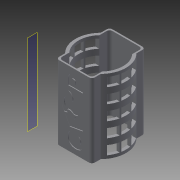
# Autodesk Inventor part: Lattice
Saved by Autodesk Inventor 2013 (Build 170138000, 138)
## iProperties
Created: 2014-07-03
Part Number: Lattice
Material: Genérico
Document SubType Name: Chapa
Designer: Administrador
Density: 1 g/cm^3
Sheet Metal Rule: Por defecto_mm
Author: Administrador
Autodesk Inventor part; units mm, degrees
ref_plane "YZ Plane" through (0, 0, 0) normal (1, 0, 0) x (0, 1, 0)
ref_plane "XZ Plane" through (0, 0, 0) normal (0, 1, 0) x (-1, 0, 0)
ref_plane "XY Plane" through (0, 0, 0) normal (0, 0, 1) x (1, 0, 0)
sketch "Boceto2" plane through (0, 0, 0) normal (0, 0, 1) x (1, 0, 0)
  line L0 (-11.1, -17.1) -> (11.1, -17.1)
  line L1 (11.1, 17.1) -> (-11.1, 17.1)
  line L2 (-11.1, -17.1) -> (11.1, 17.1) construction
  line L3 (11.1, -17.1) -> (-11.1, 17.1) construction
  arc A0 (-12.1, 12.083) -> (-12.1, -12.083) centre (0, 0) ccw
  arc A1 (12.1, -12.083) -> (12.1, 12.083) centre (0, 0) ccw
  line L4 (11.1, -17.1) -> (11.1, -13.0077)
  line L5 (11.1, 13.0077) -> (11.1, 17.1)
  line L6 (-11.1, 17.1) -> (-11.1, 13.0077)
  line L7 (-11.1, -13.0077) -> (-11.1, -17.1)
  line L8 (-44.1235, -12.996) -> (-27.2515, -12.996)
  line L9 (-27.2515, 12.996) -> (-44.1235, 12.996)
  line L10 (-44.1235, -12.996) -> (-27.2515, 12.996) construction
  line L11 (-27.2515, -12.996) -> (-44.1235, 12.996) construction
  arc A2 (-44.1235, 9.8858) -> (-44.1235, -9.8858) centre (-35.6875, 0) ccw
  arc A3 (-27.2515, -9.8858) -> (-27.2515, 9.8858) centre (-35.6875, 0) ccw
  line L12 (-27.2515, -12.996) -> (-27.2515, -9.8858)
  line L13 (-27.2515, 9.8858) -> (-27.2515, 12.996)
  line L14 (-44.1235, 12.996) -> (-44.1235, 9.8858)
  line L15 (-44.1235, -9.8858) -> (-44.1235, -12.996)
  line L16 (-12.1, -18.1) -> (12.1, -18.1)
  line L17 (12.1, 18.1) -> (-12.1, 18.1)
  line L18 (-12.1, -18.1) -> (12.1, 18.1) construction
  line L19 (12.1, -18.1) -> (-12.1, 18.1) construction
  line L20 (-12.1, 18.1) -> (-12.1, 12.083)
  line L21 (-12.1, -12.083) -> (-12.1, -18.1)
  line L22 (12.1, -18.1) -> (12.1, -12.083)
  line L23 (12.1, 12.083) -> (12.1, 18.1)
  arc A4 (-8.2215, 12.6656) -> (-8.392, 12.5533) centre (0, 0) ccw
  arc A5 (8.392, 12.5533) -> (8.2215, 12.6656) centre (0, 0) ccw
  arc A6 (-11.1, 10.2372) -> (-11.1, -10.2372) centre (0, 0) ccw
  arc A7 (-8.392, -12.5533) -> (-8.2215, -12.6656) centre (0, 0) ccw
  arc A8 (8.2215, -12.6656) -> (8.392, -12.5533) centre (0, 0) ccw
  arc A9 (11.1, -10.2372) -> (11.1, 10.2372) centre (0, 0) ccw
  line L24 (11.1, 12.996) -> (11.1, 10.2372)
  line L25 (11.1, -10.2372) -> (11.1, -12.996)
  line L26 (-11.1, 12.996) -> (-11.1, 10.2372)
  line L27 (-11.1, -10.2372) -> (-11.1, -12.996)
  dimension "d4" = 22.2
  dimension "d5" = 34.2
  dimension "d6" = 16.872
  dimension "d7" = 25.992
  dimension "d9" = 24.2
  dimension "d10" = 36.2
  constraints: 56 end point, 20 point on circle, 15 parallel, 10 centre point, 8 point on line, 6 midpoint, 6 perpendicular, 3 horizontal
  measures "d4" distance of L1.end L1.start
  measures "d5" distance of L1.start L0.end
  measures "d6" distance of L9.end L9.start
  measures "d7" distance of L9.start L8.end
  measures "d9" distance of L17.end L17.start
  measures "d10" distance of L17.start L16.end
extrude "Extrusión1" add sketch "Boceto2" along normal blind 50 contours L20 L17 L23 A1 L22 L16 L21 A0
sketch "Boceto3" plane through (0, 0, 0) normal (0, 0, -1) x (-1, 0, 0)
  line L0 (24.6329, -16.764) -> (46.8329, -16.764)
  line L1 (46.8329, 17.436) -> (24.6329, 17.436)
  line L2 (46.8329, -16.764) -> (46.8329, -12.6716)
  line L3 (46.8329, 13.3437) -> (46.8329, 17.436)
  line L4 (24.6329, 17.436) -> (24.6329, 13.3437)
  line L5 (24.6329, -12.6716) -> (24.6329, -16.764)
  arc A0 (24.6329, 10.5732) -> (24.6329, -9.9011) centre (35.7329, 0.336) ccw
  arc A1 (46.8329, -9.9011) -> (46.8329, 10.5732) centre (35.7329, 0.336) ccw
  line L6 (46.8329, 13.332) -> (46.8329, 10.5732)
  line L7 (46.8329, -9.9011) -> (46.8329, -12.66)
  line L8 (24.6329, 13.332) -> (24.6329, 10.5732)
  line L9 (24.6329, -9.9011) -> (24.6329, -12.66)
  line L10 (-11.1, 17.1) -> (11.1, 17.1)
  line L11 (11.1, -17.1) -> (-11.1, -17.1)
  line L12 (-11.1, 17.1) -> (11.1, -17.1) construction
  line L13 (11.1, 17.1) -> (-11.1, -17.1) construction
  line L14 (11.1, 17.1) -> (11.1, 10.2372)
  line L15 (11.1, -10.2372) -> (11.1, -17.1)
  arc A2 (-11.1, 10.2372) -> (-11.1, -10.2372) centre (0, 0) ccw
  arc A3 (11.1, -10.2372) -> (11.1, 10.2372) centre (0, 0) ccw
  line L16 (-11.1, -17.1) -> (-11.1, -10.2372)
  line L17 (-11.1, 10.2372) -> (-11.1, 17.1)
  dimension "d13" = 22.2
  dimension "d14" = 34.2
  dimension "d15" = 22.2
  dimension "d16" = 34.2
  constraints: 36 end point, 10 parallel, 8 point on circle, 4 centre point, 4 perpendicular, 2 horizontal, 2 midpoint
  measures "d13" distance of L1.end L1.start
  measures "d14" distance of L1.start L0.end
  measures "d15" distance of L11.start L11.end
  measures "d16" distance of L10.end L11.start
extrude "Extrusión2" cut sketch "Boceto3" against normal through all
ref_plane "Plano de trabajo1" through (-31.35, -18.1, 0) normal (-1, 0, 0) x (0, 0, 1)
sketch "Boceto4" plane through (-31.35, -18.1, 0) normal (-1, 0, 0) x (0, 0, 1)
  line L0 (0, 6.017) -> (0, 30.183) projected
  line L1 (0, 36.2) -> (0, 30.183) projected
  line L2 (0, 30.183) -> (50, 30.183) projected
  line L3 (0, 6.017) -> (50, 6.017) projected
  line L4 (50, 6.017) -> (50, 30.183) projected
  line L5 (2.0442, 28.2647) -> (8.0442, 28.2647)
  line L6 (8.0442, 28.2647) -> (8.0442, 22.2647)
  line L7 (8.0442, 22.2647) -> (2.0442, 22.2647)
  line L8 (2.0442, 22.2647) -> (2.0442, 28.2647)
  line L9 (12.0442, 28.2647) -> (18.0442, 28.2647)
  line L10 (18.0442, 28.2647) -> (18.0442, 22.2647)
  line L11 (18.0442, 22.2647) -> (12.0442, 22.2647)
  line L12 (12.0442, 22.2647) -> (12.0442, 28.2647)
  line L13 (22.0442, 28.2647) -> (28.0442, 28.2647)
  line L14 (28.0442, 28.2647) -> (28.0442, 22.2647)
  line L15 (28.0442, 22.2647) -> (22.0442, 22.2647)
  line L16 (22.0442, 22.2647) -> (22.0442, 28.2647)
  line L17 (32.0442, 28.2647) -> (38.0442, 28.2647)
  line L18 (38.0442, 28.2647) -> (38.0442, 22.2647)
  line L19 (38.0442, 22.2647) -> (32.0442, 22.2647)
  line L20 (32.0442, 22.2647) -> (32.0442, 28.2647)
  line L21 (42.0442, 28.2647) -> (48.0442, 28.2647)
  line L22 (48.0442, 28.2647) -> (48.0442, 22.2647)
  line L23 (48.0442, 22.2647) -> (42.0442, 22.2647)
  line L24 (42.0442, 22.2647) -> (42.0442, 28.2647)
  line L25 (2.0442, 21.2647) -> (8.0442, 21.2647)
  line L26 (8.0442, 21.2647) -> (8.0442, 15.2647)
  line L27 (8.0442, 15.2647) -> (2.0442, 15.2647)
  line L28 (2.0442, 15.2647) -> (2.0442, 21.2647)
  line L29 (12.0442, 21.2647) -> (18.0442, 21.2647)
  line L30 (18.0442, 21.2647) -> (18.0442, 15.2647)
  line L31 (18.0442, 15.2647) -> (12.0442, 15.2647)
  line L32 (12.0442, 15.2647) -> (12.0442, 21.2647)
  line L33 (22.0442, 21.2647) -> (28.0442, 21.2647)
  line L34 (28.0442, 21.2647) -> (28.0442, 15.2647)
  line L35 (28.0442, 15.2647) -> (22.0442, 15.2647)
  line L36 (22.0442, 15.2647) -> (22.0442, 21.2647)
  line L37 (32.0442, 21.2647) -> (38.0442, 21.2647)
  line L38 (38.0442, 21.2647) -> (38.0442, 15.2647)
  line L39 (38.0442, 15.2647) -> (32.0442, 15.2647)
  line L40 (32.0442, 15.2647) -> (32.0442, 21.2647)
  line L41 (42.0442, 21.2647) -> (48.0442, 21.2647)
  line L42 (48.0442, 21.2647) -> (48.0442, 15.2647)
  line L43 (48.0442, 15.2647) -> (42.0442, 15.2647)
  line L44 (42.0442, 15.2647) -> (42.0442, 21.2647)
  line L45 (2.0442, 14.2647) -> (8.0442, 14.2647)
  line L46 (8.0442, 14.2647) -> (8.0442, 8.2647)
  line L47 (8.0442, 8.2647) -> (2.0442, 8.2647)
  line L48 (2.0442, 8.2647) -> (2.0442, 14.2647)
  line L49 (12.0442, 14.2647) -> (18.0442, 14.2647)
  line L50 (18.0442, 14.2647) -> (18.0442, 8.2647)
  line L51 (18.0442, 8.2647) -> (12.0442, 8.2647)
  line L52 (12.0442, 8.2647) -> (12.0442, 14.2647)
  line L53 (22.0442, 14.2647) -> (28.0442, 14.2647)
  line L54 (28.0442, 14.2647) -> (28.0442, 8.2647)
  line L55 (28.0442, 8.2647) -> (22.0442, 8.2647)
  line L56 (22.0442, 8.2647) -> (22.0442, 14.2647)
  line L57 (32.0442, 14.2647) -> (38.0442, 14.2647)
  line L58 (38.0442, 14.2647) -> (38.0442, 8.2647)
  line L59 (38.0442, 8.2647) -> (32.0442, 8.2647)
  line L60 (32.0442, 8.2647) -> (32.0442, 14.2647)
  line L61 (42.0442, 14.2647) -> (48.0442, 14.2647)
  line L62 (48.0442, 14.2647) -> (48.0442, 8.2647)
  line L63 (48.0442, 8.2647) -> (42.0442, 8.2647)
  line L64 (42.0442, 8.2647) -> (42.0442, 14.2647)
  point P0 (0, 18.1)
  dimension "d21" = 6
  dimension "d22" = 6
  dimension "d25" = 10
  dimension "d28" = 7
  constraints: 120 end point, 2 horizontal, 2 parallel, 1 perpendicular, 1 vertical, 112 other
  measures "d21" distance of L6.end L7.end
  measures "d22" distance of L5.end L6.end
  measures "d25" distance of L5.start L9.start
  measures "d28" distance of L5.start L25.start
extrude "Extrusión3" cut sketch "Boceto4" against normal through all contours L5 L6 L7 L8 | L9 L10 L11 L12 | L13 L14 L15 L16 | L17 L18 L19 L20 | L21 L22 L23 L24 | L25 L26 L27 L28 | L29 L30 L31 L32 | L33 L34 L35 L36 | L37 L38 L39 L40 | L41 L42 L43 L44 | L45 L46 L47 L48 | L49 L50 L51 L52 | L53 L54 L55 L56 | L57 L58 L59 L60 | L61 L62 L63 L64
fillet "Empalme1" radius 2 4 edges at (-11.1, 17.1, 25) (-11.1, -17.1, 25) (11.1, 17.1, 25) (11.1, -17.1, 25)
fillet "Empalme2" radius 2 4 edges at (-12.1, -18.1, 25) (-12.1, 18.1, 25) (12.1, 18.1, 25) (12.1, -18.1, 25)
sketch "Boceto5" plane through (-10.1, -18.1, 0) normal (0, -1, 0) x (1, 0, 0)
  line L0 (16.362, 3.0305) -> (5.973, 3.0305) construction
  line L1 (5.973, 3.0305) -> (5.973, 30.3224) construction
  line L2 (5.973, 30.3224) -> (16.362, 30.3224) construction
  line L3 (16.362, 30.3224) -> (16.362, 3.0305) construction
  line L4 (16.0941, 16.2085) -> (12.8478, 22.3142)
  line L5 (7.0479, 14.6134) -> (3.8014, 20.7191)
  line L6 (5.616, 13.5808) -> (5.616, 17.3064) construction
  line L7 (16.0941, 16.2085) -> (7.0479, 14.6134)
  line L8 (16.1742, 37.4402) -> (6.1742, 37.4402) construction
  line L9 (6.1742, 37.4402) -> (6.1742, 46.4759) construction
  line L10 (6.1742, 46.4759) -> (16.1742, 46.4759) construction
  line L11 (16.1742, 46.4759) -> (16.1742, 37.4402) construction
  line L12 (12.3094, 23.3269) -> (12.309, 23.3277)
  ellipse E0 centre (9.1564, 29.2567) end of major axis (12.3118, 23.3282) minor radius 3.4628 (12.3094, 23.3269) -> (6.0035, 35.1865) ccw
  line L13 (8.8079, 29.9125) -> (6.0037, 35.1867) construction
  ellipse E1 centre (7.4058, 32.5496) end of major axis (8.8079, 29.9125) minor radius 1.3012 (8.8076, 29.9124) -> (6.0035, 35.1865) ccw
  line L14 (10.5528, 21.9095) -> (12.8478, 22.3142)
  line L15 (3.8014, 20.7191) -> (6.484, 21.1921)
  line L16 (9.8284, 22.8903) -> (12.3118, 23.3282)
  line L17 (3.2625, 21.7327) -> (5.5901, 22.1431)
  ellipse E2 centre (7.9717, 22.2035) end of major axis (5.3463, 23.7267) minor radius 1.6776 (9.8284, 22.8903) -> (5.5901, 22.1431) ccw
  line L18 (3.2625, 21.7327) -> (1.5614, 24.932)
  line L19 (1.5614, 24.932) -> (3.9638, 25.3556)
  ellipse E3 centre (7.9717, 25.4869) end of major axis (4.3959, 30.9153) minor radius 3.6119 (8.8076, 29.9124) -> (3.9638, 25.3556) ccw
  ellipse E4 centre (7.9717, 22.2035) end of major axis (5.3463, 23.7267) minor radius 1.6776 (6.484, 21.1921) -> (10.5528, 21.9095) ccw
  spline S0 degree 2 poles (16.362, 8.379) (16.362, 6.1261) (13.6391, 3.4843) (11.1756, 3.4843) knots 0 0 0 1 2 2 2
  spline S1 degree 2 poles (11.1756, 3.4843) (8.8012, 3.4843) (5.973, 6.1342) (5.973, 8.3871) knots 0 0 0 1 2 2 2
  spline S2 degree 2 poles (5.973, 8.3871) (5.973, 8.9786) (6.1108, 9.9349) (6.2242, 10.3725) knots 0 0 0 1 2 2 2
  spline S3 degree 2 poles (6.2242, 10.3725) (6.3296, 10.7128) (6.678, 11.5151) (6.8077, 11.7663) knots 0 0 0 1 2 2 2
  line L20 (6.8077, 11.7663) -> (9.1902, 11.7663)
  line L21 (9.1902, 11.7663) -> (9.1902, 11.5151)
  spline S4 degree 2 poles (9.1902, 11.5151) (9.0281, 11.3287) (8.5743, 10.7777) (8.3636, 10.4292) knots 0 0 0 1 2 2 2
  spline S5 degree 2 poles (8.3636, 10.4292) (8.1448, 10.0808) (7.845, 9.2461) (7.845, 8.7842) knots 0 0 0 1 2 2 2
  spline S6 degree 2 poles (7.845, 8.7842) (7.845, 8.2412) (8.1853, 7.3417) (8.6148, 6.9284) knots 0 0 0 1 2 2 2
  spline S7 degree 2 poles (8.6148, 6.9284) (8.9957, 6.5556) (10.3004, 6.0775) (11.1837, 6.0775) knots 0 0 0 1 2 2 2
  spline S8 degree 2 poles (11.1837, 6.0775) (12.1156, 6.0775) (13.3879, 6.5718) (13.7769, 6.977) knots 0 0 0 1 2 2 2
  spline S9 degree 2 poles (13.7769, 6.977) (14.1578, 7.366) (14.49, 8.3222) (14.49, 8.8004) knots 0 0 0 1 2 2 2
  spline S10 degree 2 poles (14.49, 8.8004) (14.49, 9.2947) (14.1578, 10.1942) (13.9552, 10.5021) knots 0 0 0 1 2 2 2
  spline S11 degree 2 poles (13.9552, 10.5021) (13.7526, 10.8425) (13.3231, 11.353) (13.1529, 11.5394) knots 0 0 0 1 2 2 2
  line L22 (13.1529, 11.5394) -> (13.1529, 11.7663)
  line L23 (13.1529, 11.7663) -> (15.503, 11.7663)
  spline S12 degree 2 poles (15.503, 11.7663) (15.6326, 11.4908) (15.9568, 10.7696) (16.0702, 10.3806) knots 0 0 0 1 2 2 2
  spline S13 degree 2 poles (16.0702, 10.3806) (16.2161, 9.9106) (16.362, 9.0921) (16.362, 8.379) knots 0 0 0 1 2 2 2
  spline S14 degree 2 poles (9.3266, 46.1679) (10.0235, 46.1679) (11.2877, 45.7222) (11.7091, 45.3089) knots 0 0 0 1 2 2 2
  spline S15 degree 2 poles (11.7091, 45.3089) (11.9765, 45.0577) (12.4141, 44.4418) (12.5681, 44.0772) knots 0 0 0 1 2 2 2
  spline S16 degree 2 poles (12.5681, 44.0772) (12.722, 43.7044) (12.9003, 42.8373) (12.9003, 42.3024) knots 0 0 0 1 2 2 2
  line L24 (12.9003, 42.3024) -> (12.9003, 40.9896)
  line L25 (12.9003, 40.9896) -> (16.1742, 40.9896)
  line L26 (16.1742, 40.9896) -> (16.1742, 38.4775)
  line L27 (16.1742, 38.4775) -> (6.1742, 38.4775)
  line L28 (6.1742, 38.4775) -> (6.1742, 42.3592)
  spline S17 degree 2 poles (6.1742, 42.3592) (6.1742, 43.2182) (6.4903, 44.4742) (6.8306, 44.9848) knots 0 0 0 1 2 2 2
  spline S18 degree 2 poles (6.8306, 44.9848) (7.2115, 45.552) (8.4595, 46.1679) (9.3266, 46.1679) knots 0 0 0 1 2 2 2
  spline S19 degree 2 poles (9.3914, 43.5909) (8.9619, 43.5909) (8.3541, 43.1857) (8.2407, 42.9102) knots 0 0 0 1 2 2 2
  spline S20 degree 2 poles (8.2407, 42.9102) (8.0867, 42.5536) (8.0381, 41.9054) (8.0381, 41.3462) knots 0 0 0 1 2 2 2
  line L29 (8.0381, 41.3462) -> (8.0381, 40.9896)
  line L30 (8.0381, 40.9896) -> (11.0365, 40.9896)
  line L31 (11.0365, 40.9896) -> (11.0365, 41.1679)
  spline S21 degree 2 poles (11.0365, 41.1679) (11.0365, 41.5164) (11.0202, 42.1485) (10.9797, 42.3835) knots 0 0 0 1 2 2 2
  spline S22 degree 2 poles (10.9797, 42.3835) (10.9473, 42.5861) (10.7528, 43.0318) (10.6313, 43.1533) knots 0 0 0 1 2 2 2
  spline S23 degree 2 poles (10.6313, 43.1533) (10.3882, 43.4126) (9.8452, 43.5909) (9.3914, 43.5909) knots 0 0 0 1 2 2 2
  point P0 (10.1, 0)
  point P1 (10.2553, 24.9935)
  point P2 (9.3115, 25.0171)
  point P3 (16.0941, 25.3943)
  point P4 (16.0941, 36.6277)
  constraints: 24 end point, 2 point on line, 26 other
emboss "Repujado1" sketch "Boceto5" operation cut depth 0.5 direction (0, 1, 0)
sketch "Boceto6" plane through (-10.1, 18.1, 0) normal (0, 1, 0) x (1, 0, 0)
  line L0 (3.7797, -3.1095) -> (14.1687, -3.1095) construction
  line L1 (14.1687, -3.1095) -> (14.1687, -30.4014) construction
  line L2 (14.1687, -30.4014) -> (3.7797, -30.4014) construction
  line L3 (3.7797, -30.4014) -> (3.7797, -3.1095) construction
  line L4 (4.0475, -16.2875) -> (13.0938, -14.6924)
  line L5 (14.5257, -13.6598) -> (14.5257, -17.3854) construction
  line L6 (4.0475, -16.2875) -> (7.2939, -22.3932)
  line L7 (13.0938, -14.6924) -> (16.3402, -20.7981)
  line L8 (9.5889, -21.9885) -> (7.2939, -22.3932)
  ellipse E0 centre (12.17, -22.2825) end of major axis (14.7954, -23.8057) minor radius 1.6776 (13.6576, -21.2711) -> (9.5889, -21.9885) ccw
  line L9 (3.9674, -37.5192) -> (13.9674, -37.5192) construction
  line L10 (13.9674, -37.5192) -> (13.9674, -46.5549) construction
  line L11 (13.9674, -46.5549) -> (3.9674, -46.5549) construction
  line L12 (3.9674, -46.5549) -> (3.9674, -37.5192) construction
  line L13 (10.3133, -22.9693) -> (7.8299, -23.4072)
  ellipse E1 centre (12.17, -22.2825) end of major axis (14.7954, -23.8057) minor radius 1.6776 (10.3133, -22.9693) -> (14.5515, -22.2221) ccw
  line L14 (7.8323, -23.4059) -> (7.8327, -23.4067)
  ellipse E2 centre (12.17, -25.5659) end of major axis (15.7458, -30.9944) minor radius 3.6119 (11.334, -29.9914) -> (16.1778, -25.4346) ccw
  ellipse E3 centre (10.9852, -29.3357) end of major axis (7.8299, -23.4072) minor radius 3.4628 (7.8323, -23.4059) -> (14.1382, -35.2655) ccw
  line L15 (11.3338, -29.9915) -> (14.138, -35.2657) construction
  ellipse E4 centre (12.7359, -32.6286) end of major axis (11.3338, -29.9915) minor radius 1.3012 (11.334, -29.9914) -> (14.1382, -35.2655) ccw
  line L16 (18.5803, -25.011) -> (16.1778, -25.4346)
  line L17 (16.8792, -21.8117) -> (14.5515, -22.2221)
  line L18 (16.8792, -21.8117) -> (18.5803, -25.011)
  line L19 (16.3402, -20.7981) -> (13.6576, -21.2711)
  spline S0 degree 2 poles (3.7797, -8.458) (3.7797, -6.2051) (6.5025, -3.5633) (8.9661, -3.5633) knots 0 0 0 1 2 2 2
  spline S1 degree 2 poles (8.9661, -3.5633) (11.3405, -3.5633) (14.1687, -6.2132) (14.1687, -8.4661) knots 0 0 0 1 2 2 2
  spline S2 degree 2 poles (14.1687, -8.4661) (14.1687, -9.0577) (14.0309, -10.0139) (13.9175, -10.4515) knots 0 0 0 1 2 2 2
  spline S3 degree 2 poles (13.9175, -10.4515) (13.8121, -10.7919) (13.4636, -11.5941) (13.334, -11.8453) knots 0 0 0 1 2 2 2
  line L20 (13.334, -11.8453) -> (10.9515, -11.8453)
  line L21 (10.9515, -11.8453) -> (10.9515, -11.5941)
  spline S4 degree 2 poles (10.9515, -11.5941) (11.1136, -11.4077) (11.5674, -10.8567) (11.7781, -10.5082) knots 0 0 0 1 2 2 2
  spline S5 degree 2 poles (11.7781, -10.5082) (11.9969, -10.1598) (12.2967, -9.3251) (12.2967, -8.8632) knots 0 0 0 1 2 2 2
  spline S6 degree 2 poles (12.2967, -8.8632) (12.2967, -8.3202) (11.9564, -7.4207) (11.5269, -7.0074) knots 0 0 0 1 2 2 2
  spline S7 degree 2 poles (11.5269, -7.0074) (11.146, -6.6346) (9.8413, -6.1565) (8.958, -6.1565) knots 0 0 0 1 2 2 2
  spline S8 degree 2 poles (8.958, -6.1565) (8.026, -6.1565) (6.7538, -6.6509) (6.3648, -7.056) knots 0 0 0 1 2 2 2
  spline S9 degree 2 poles (6.3648, -7.056) (5.9839, -7.445) (5.6517, -8.4013) (5.6517, -8.8794) knots 0 0 0 1 2 2 2
  spline S10 degree 2 poles (5.6517, -8.8794) (5.6517, -9.3737) (5.9839, -10.2732) (6.1865, -10.5812) knots 0 0 0 1 2 2 2
  spline S11 degree 2 poles (6.1865, -10.5812) (6.3891, -10.9215) (6.8186, -11.432) (6.9888, -11.6184) knots 0 0 0 1 2 2 2
  line L22 (6.9888, -11.6184) -> (6.9888, -11.8453)
  line L23 (6.9888, -11.8453) -> (4.6387, -11.8453)
  spline S12 degree 2 poles (4.6387, -11.8453) (4.509, -11.5698) (4.1849, -10.8486) (4.0714, -10.4596) knots 0 0 0 1 2 2 2
  spline S13 degree 2 poles (4.0714, -10.4596) (3.9256, -9.9896) (3.7797, -9.1711) (3.7797, -8.458) knots 0 0 0 1 2 2 2
  spline S14 degree 2 poles (10.8151, -46.2469) (10.1182, -46.2469) (8.854, -45.8012) (8.4326, -45.3879) knots 0 0 0 1 2 2 2
  spline S15 degree 2 poles (8.4326, -45.3879) (8.1652, -45.1367) (7.7276, -44.5208) (7.5736, -44.1562) knots 0 0 0 1 2 2 2
  spline S16 degree 2 poles (7.5736, -44.1562) (7.4196, -43.7834) (7.2413, -42.9163) (7.2413, -42.3814) knots 0 0 0 1 2 2 2
  line L24 (7.2413, -42.3814) -> (7.2413, -41.0686)
  line L25 (7.2413, -41.0686) -> (3.9674, -41.0686)
  line L26 (3.9674, -41.0686) -> (3.9674, -38.5565)
  line L27 (3.9674, -38.5565) -> (13.9674, -38.5565)
  line L28 (13.9674, -38.5565) -> (13.9674, -42.4382)
  spline S17 degree 2 poles (13.9674, -42.4382) (13.9674, -43.2972) (13.6514, -44.5532) (13.311, -45.0638) knots 0 0 0 1 2 2 2
  spline S18 degree 2 poles (13.311, -45.0638) (12.9302, -45.631) (11.6822, -46.2469) (10.8151, -46.2469) knots 0 0 0 1 2 2 2
  spline S19 degree 2 poles (10.7503, -43.6699) (11.1798, -43.6699) (11.7875, -43.2647) (11.901, -42.9892) knots 0 0 0 1 2 2 2
  spline S20 degree 2 poles (11.901, -42.9892) (12.055, -42.6327) (12.1036, -41.9844) (12.1036, -41.4252) knots 0 0 0 1 2 2 2
  line L29 (12.1036, -41.4252) -> (12.1036, -41.0686)
  line L30 (12.1036, -41.0686) -> (9.1052, -41.0686)
  line L31 (9.1052, -41.0686) -> (9.1052, -41.2469)
  spline S21 degree 2 poles (9.1052, -41.2469) (9.1052, -41.5954) (9.1214, -42.2275) (9.1619, -42.4625) knots 0 0 0 1 2 2 2
  spline S22 degree 2 poles (9.1619, -42.4625) (9.1943, -42.6651) (9.3888, -43.1108) (9.5104, -43.2323) knots 0 0 0 1 2 2 2
  spline S23 degree 2 poles (9.5104, -43.2323) (9.7535, -43.4917) (10.2965, -43.6699) (10.7503, -43.6699) knots 0 0 0 1 2 2 2
  point P0 (10.1, 0)
  point P1 (10.0417, -0.079)
  point P2 (4.0475, -36.7067)
  point P3 (9.8864, -25.0725)
  point P4 (10.8301, -25.0961)
  point P5 (4.0475, -25.4733)
  constraints: 24 end point, 2 point on line, 26 other
emboss "Repujado2" sketch "Boceto6" operation cut depth 0.5 direction (0, -1, 0)
equation "\"Tamaño_de_radio_de_Jacobi\" = Radio_pliegue"
equation "\"Radio_pliegue\" = Grosor"
equation "\"Anchura_desahogo_plegado\" = Grosor"
equation "\"Profundidad_desahogo_plegado\" = 0.5 * Grosor"
equation "\"Tamaño_destalonado\" = 4 * Grosor"
equation "\"Remanente_mínimo\" = 2 * Grosor"
equation "\"Radiodetransición\" = Radio_pliegue"
equation "\"TamañoSeparación\" = Grosor"
equation "\"Grosor\" = 0.5"
